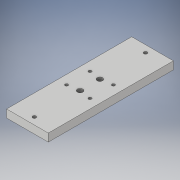
# Autodesk Inventor part: Platform A
Saved by Autodesk Inventor 2019.4 (Build 234330000, 330)
## iProperties
Created: 2021-01-08
Part Number: Platform A
Material: Generic
Document SubType Name: Modeling
Designer: caleb
Density: 1 g/cm^3
Appearance: Default
Author: caleb
Autodesk Inventor part; units mm, degrees
ref_plane "YZ Plane" through (0, 0, 0) normal (1, 0, 0) x (0, 1, 0)
ref_plane "XZ Plane" through (0, 0, 0) normal (0, 1, 0) x (-1, 0, 0)
ref_plane "XY Plane" through (0, 0, 0) normal (0, 0, 1) x (1, 0, 0)
sketch "Sketch1" plane through (0, 0, 0) normal (0, 1, 0) x (-1, 0, 0)
  line L0 (-14.9987, 44.9961) -> (14.9987, 44.9961)
  line L1 (14.9987, 44.9961) -> (14.9987, -44.9961)
  line L2 (14.9987, -44.9961) -> (-14.9987, -44.9961)
  line L3 (-14.9987, -44.9961) -> (-14.9987, 44.9961)
  line L4 (-14.9987, 44.9961) -> (14.9987, -44.9961) construction
  line L5 (14.9987, 44.9961) -> (-14.9987, -44.9961) construction
  point P0 (0, 0)
  dimension "d0" = 89.9922
  dimension "d1" = 29.9974
  constraints: 12 end point, 2 midpoint, 2 parallel, 1 horizontal, 1 perpendicular
  measures "d0" distance of L0.end L1.end
  measures "d1" distance of L0.start L0.end
extrude "Extrusion1" add sketch "Sketch1" along normal blind 6.35
sketch "Sketch5" plane through (0, 6.35, 0) normal (0, 1, 0) x (1, 0, 0)
  circle A0 centre (0, -39.9923) radius 1.4986
  circle A1 centre (0, 39.9923) radius 1.4986
  line L0 (-14.9987, -44.9961) -> (14.9987, -44.9961) projected
  line L1 (14.9987, 44.9961) -> (-14.9987, 44.9961) projected
  point P0 (0, 0)
  dimension "d33" = 2.9972
  dimension "d34" = 2.9972
  dimension "d35" = 5.0038
  dimension "d36" = 5.0038
  constraints: 2 centre point
  measures "d33" diameter of A0
  measures "d34" diameter of A1
  measures "d35" distance from line of L0 A0.centre
  measures "d36" distance from line of L1 A1.centre
hole "Hole2" at (0, 6.35, 39.9923) at (0, 6.35, -39.9923) direction (0, -1, 0) diameter 2.4638 depth 5.588 tip angle 118
sketch "Sketch6" plane through (0, 0, 0) normal (0, -1, 0) x (1, 0, 0)
  circle A0 centre (0, 7.1) radius 2.0701
  circle A1 centre (0, -7.1) radius 2.0701
  point P0 (0, 0)
  dimension "d44" = 4.1402
  dimension "d45" = 7.1
  dimension "d46" = 4.1402
  dimension "d47" = 7.1
  constraints: 2 centre point
  measures "d44" diameter of A0
  measures "d45" distance of point (0, 0) A0.centre
  measures "d46" diameter of A1
  measures "d47" distance of point (0, 0) A1.centre
hole "Hole3" at (0, 0, -7.1) at (0, 0, 7.1) direction (0, 1, 0) diameter 3.9624 depth 13.6144 tip angle 118 thread size "10-32 UNF" class "2B" standard "ANSI Unified Screw Threads"
sketch "Sketch7" plane through (0, 6.35, 0) normal (0, 1, 0) x (1, 0, 0)
  circle A0 centre (-8.4201, -8.4201) radius 1.4986
  line L0 (-14.9987, 44.9961) -> (-14.9987, -44.9961)
  line L1 (-14.9987, -44.9961) -> (14.9987, -44.9961)
  circle A1 centre (-8.4201, 8.4201) radius 1.4986
  circle A2 centre (8.4201, -8.4201) radius 1.4986
  circle A3 centre (8.4201, 8.4201) radius 1.4986
  point P0 (0, 0)
  dimension "d62" = 2.9972
  dimension "d64" = 8.4201
  dimension "d57" = 16.8402
  dimension "d56" = 16.8402
  dimension "d63" = 8.4201
  constraints: 4 centre point, 4 end point, 1 horizontal, 1 vertical, 6 other
  measures "d62" diameter of A0
  measures "d64" horizontal distance of A0.centre point (0, 0)
  measures "d57" distance of A0.centre A1.centre
  measures "d56" distance of A0.centre A2.centre
  measures "d63" horizontal distance of point (0, 0) A0.centre
hole "Hole4" at (8.4201, 6.35, -8.4201) at (-8.4201, 6.35, -8.4201) at (-8.4201, 6.35, 8.4201) at (8.4201, 6.35, 8.4201) direction (0, -1, 0) diameter 2.159 depth 5.588 tip angle 118
chamfer "Chamfer2" distance 0.7112 angle 45 4 edges at (14.9987, 0, 0) (0, 0, 44.9961) (-14.9987, 0, 0) (0, 0, -44.9961)
body "Solid1"
